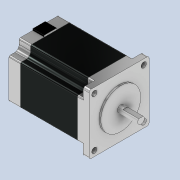
# Autodesk Inventor part: Nema 23 76.5mm Stepper Motor
Saved by Autodesk Inventor 2022 (Build 260153000, 153)
## iProperties
Created: 2021-10-18
Part Number: Nema 23 76.5mm Stepper Motor
Material: Generic
Document SubType Name: Modeling
Designer: Coy
Density: 1 g/cm^3
Appearance: Chrome - Polished
Author: Coy
Autodesk Inventor part; units mm, degrees
ref_plane "YZ Plane" through (0, 0, 0) normal (1, 0, 0) x (0, 1, 0)
ref_plane "XZ Plane" through (0, 0, 0) normal (0, 1, 0) x (-1, 0, 0)
ref_plane "XY Plane" through (0, 0, 0) normal (0, 0, 1) x (1, 0, 0)
sketch "Sketch1" plane through (0, 0, 0) normal (1, 0, 0) x (0, 1, 0)
  line L0 (2, 0) -> (55.3, 0)
  line L1 (57.3, -2) -> (57.3, -55.3)
  line L2 (55.3, -57.3) -> (2, -57.3)
  line L3 (0, -55.3) -> (0, -2)
  arc A0 (57.3, -2) -> (55.3, 0) centre (55.3, -2) ccw
  arc A1 (55.3, -57.3) -> (57.3, -55.3) centre (55.3, -55.3) ccw
  arc A2 (0, -55.3) -> (2, -57.3) centre (2, -55.3) ccw
  arc A3 (2, 0) -> (0, -2) centre (2, -2) ccw
  line L4 (52.22, -5.08) -> (5.08, -5.08) construction
  line L5 (5.08, -5.08) -> (5.08, -52.22) construction
  line L6 (5.08, -52.22) -> (52.22, -52.22) construction
  line L7 (52.22, -52.22) -> (52.22, -5.08) construction
  line L8 (52.22, -5.08) -> (57.3, -5.08) construction
  line L9 (52.22, -5.08) -> (52.22, 0) construction
  line L10 (5.08, -52.22) -> (0, -52.22) construction
  line L11 (5.08, -52.22) -> (5.08, -57.3) construction
  circle A4 centre (52.22, -5.08) radius 2.5
  circle A5 centre (52.22, -52.22) radius 2.5
  circle A6 centre (5.08, -52.22) radius 2.5
  circle A7 centre (5.08, -5.08) radius 2.5
  point P0 (0, 0)
  point P1 (57.3, -57.3)
  point P2 (57.3, 0)
  point P3 (0, -57.3)
  dimension "d0" = 57.3
  dimension "d1" = 57.3
  dimension "d2" = 2
  dimension "d3" = 2
  dimension "d4" = 5
  dimension "d5" = 5
  dimension "d6" = 5
  dimension "d7" = 5
  dimension "d8" = 47.14
  dimension "d9" = 47.14
  constraints: 24 end point, 12 point on line, 8 centre point, 8 point on circle, 8 tangent, 6 parallel, 6 perpendicular, 4 coincident, 2 equal radius, 2 horizontal
  measures "d0" distance of point (57.3, -57.3) point (0, -57.3)
  measures "d1" distance of point (57.3, 0) point (57.3, -57.3)
  measures "d2" radius of A0
  measures "d3" radius of A3
  measures "d4" diameter of A4
  measures "d5" diameter of A5
  measures "d6" diameter of A6
  measures "d7" diameter of A7
  measures "d8" distance of L4.start L4.end
  measures "d9" distance of L6.end L4.start
extrude "Extrusion1" add sketch "Sketch1" along normal blind 5.5
sketch "Sketch2" plane through (0, 0, 0) normal (-1, 0, 0) x (0, 0, 1)
  line L0 (-57.3, 2) -> (-57.3, 55.3) construction
  arc A0 (-57.3, 2) -> (-55.3, 0) centre (-55.3, 2) ccw projected
  line L1 (-2, 0) -> (-55.3, 0) construction
  arc A1 (-2, 0) -> (0, 2) centre (-2, 2) ccw projected
  line L2 (0, 55.3) -> (0, 2) construction
  arc A2 (0, 55.3) -> (-2, 57.3) centre (-2, 55.3) ccw projected
  line L3 (-55.3, 57.3) -> (-2, 57.3) construction
  arc A3 (-55.3, 57.3) -> (-57.3, 55.3) centre (-55.3, 55.3) ccw projected
  circle A4 centre (-5.08, 52.22) radius 2.5 projected
  circle A5 centre (-52.22, 52.22) radius 2.5 projected
  circle A6 centre (-52.22, 5.08) radius 2.5 projected
  circle A7 centre (-5.08, 5.08) radius 2.5 projected
  line L4 (-55.3, 57.3) -> (-2, 57.3) construction
  line L5 (-47.65, 57.3) -> (-9.65, 57.3)
  line L6 (-57.3, 2) -> (-57.3, 55.3) construction
  line L7 (-57.3, 9.65) -> (-57.3, 47.65)
  line L8 (-2, 0) -> (-55.3, 0) construction
  line L9 (-47.65, 0) -> (-9.65, 0)
  line L10 (0, 9.65) -> (0, 47.65)
  line L11 (0, 55.3) -> (0, 2) construction
  circle A8 centre (-52.22, 5.08) radius 2.5 construction
  line L12 (-52.22, 5.08) -> (-5.08, 52.22) construction
  line L13 (-28.65, 28.65) -> (-28.65, 57.3) construction
  line L14 (-28.65, 28.65) -> (-28.65, 0) construction
  line L15 (-28.65, 28.65) -> (0, 28.65) construction
  line L16 (-28.65, 28.65) -> (-57.3, 28.65) construction
  arc A9 (-51.5421, 47.65) -> (-47.6, 52.22) centre (-52.22, 52.22) ccw
  arc A10 (-9.7, 52.22) -> (-5.7579, 47.65) centre (-5.08, 52.22) ccw
  arc A11 (-5.7579, 9.65) -> (-9.7, 5.08) centre (-5.08, 5.08) ccw
  arc A12 (-47.6, 5.08) -> (-51.5421, 9.65) centre (-52.22, 5.08) ccw
  line L17 (-47.65, 57.3) -> (-47.6, 52.22)
  line L18 (-57.3, 47.65) -> (-51.5421, 47.65)
  line L19 (-9.7, 5.08) -> (-9.65, 0)
  line L20 (0, 9.65) -> (-5.7579, 9.65)
  line L21 (-9.6451, 47.6951) -> (-9.6048, 47.6952)
  line L22 (-5.7579, 47.65) -> (0, 47.65)
  line L23 (-9.65, 57.3) -> (-9.7, 52.22)
  line L24 (-9.6451, 47.6951) -> (-9.6451, 47.6549)
  line L25 (-47.6048, 9.6549) -> (-47.6452, 9.6548)
  line L26 (-51.5421, 9.65) -> (-57.3, 9.65)
  line L27 (-47.6049, 9.6951) -> (-47.6048, 9.6549)
  line L28 (-47.6, 5.08) -> (-47.65, 0)
  arc A13 (-56.05, 47.65) -> (-57.3, 46.4) centre (-56.05, 46.4) ccw
  arc A14 (-46.3876, 57.3) -> (-47.6376, 56.0377) centre (-46.3876, 56.05) ccw
  arc A15 (-9.6624, 56.0377) -> (-10.9124, 57.3) centre (-10.9124, 56.05) ccw
  arc A16 (0, 46.4) -> (-1.25, 47.65) centre (-1.25, 46.4) ccw
  arc A17 (-1.25, 9.65) -> (0, 10.9) centre (-1.25, 10.9) ccw
  arc A18 (-10.9124, 0) -> (-9.6624, 1.2623) centre (-10.9124, 1.25) ccw
  arc A19 (-47.6376, 1.2623) -> (-46.3876, 0) centre (-46.3876, 1.25) ccw
  arc A20 (-57.3, 10.9) -> (-56.05, 9.65) centre (-56.05, 10.9) ccw
  line L29 (-55.3, 57.3) -> (-2, 57.3) projected
  line L30 (-57.3, 2) -> (-57.3, 55.3) projected
  line L31 (0, 55.3) -> (0, 2) projected
  point P0 (0, 0)
  point P1 (-10.9124, 57.3)
  dimension "d12" = 38
  dimension "d13" = 38
  dimension "d14" = 38
  dimension "d15" = 38
  dimension "d16" = 2.12
  dimension "d17" = 2.12
  dimension "d18" = 2.12
  dimension "d19" = 2.12
  dimension "d20" = 2.5
  dimension "d21" = 2.5
  dimension "d22" = 2.5
  dimension "d23" = 2.5
  dimension "d24" = 2.5
  dimension "d25" = 2.5
  dimension "d26" = 2.5
  dimension "d27" = 2.5
  constraints: 42 end point, 27 point on line, 24 point on circle, 16 tangent, 12 centre point, 5 midpoint, 3 vertical, 2 horizontal
  measures "d12" distance of L5.start L5.end
  measures "d13" distance of L7.start L7.end
  measures "d14" distance of L10.end L10.start
  measures "d15" distance of L9.start L9.end
  measures "d16" radial gap between concentric circles of A5 A9
  measures "d17" radial gap between concentric circles of A4 A10
  measures "d18" radial gap between concentric circles of A7 A11
  measures "d19" radial gap between concentric circles of A6 A12
  measures "d20" diameter of A13
  measures "d21" diameter of A14
  measures "d22" diameter of A15
  measures "d23" diameter of A16
  measures "d24" diameter of A17
  measures "d25" diameter of A18
  measures "d26" diameter of A19
  measures "d27" diameter of A20
extrude "Extrusion2" add sketch "Sketch2" along normal blind 5.5 contours L10 A17 L20 A11 L19 A18 L9 A19 L28 A12 L26 A20 L7 A13 L18 A9 L17 A14 L5 A15 L23 A10 L22 A16
sketch "Sketch3" plane through (-5.5, 0, 0) normal (-1, 0, 0) x (0, 0, 1)
  line L0 (-51.5421, 47.65) -> (-56.05, 47.65) projected
  arc A0 (-56.05, 47.65) -> (-57.3, 46.4) centre (-56.05, 46.4) ccw projected
  line L1 (-57.3, 46.4) -> (-57.3, 10.9) projected
  arc A1 (-57.3, 10.9) -> (-56.05, 9.65) centre (-56.05, 10.9) ccw projected
  line L2 (-56.05, 9.65) -> (-51.5421, 9.65) projected
  arc A2 (-47.6, 5.08) -> (-51.5421, 9.65) centre (-52.22, 5.08) ccw projected
  line L3 (-47.6, 5.08) -> (-47.6376, 1.2623) projected
  arc A3 (-47.6376, 1.2623) -> (-46.3876, 0) centre (-46.3876, 1.25) ccw projected
  line L4 (-46.3876, 0) -> (-10.9124, 0) projected
  arc A4 (-10.9124, 0) -> (-9.6624, 1.2623) centre (-10.9124, 1.25) ccw projected
  line L5 (-9.6624, 1.2623) -> (-9.7, 5.08) projected
  arc A5 (-5.7579, 9.65) -> (-9.7, 5.08) centre (-5.08, 5.08) ccw projected
  line L6 (-5.7579, 9.65) -> (-1.25, 9.65) projected
  arc A6 (-1.25, 9.65) -> (0, 10.9) centre (-1.25, 10.9) ccw projected
  line L7 (0, 10.9) -> (0, 46.4) projected
  arc A7 (0, 46.4) -> (-1.25, 47.65) centre (-1.25, 46.4) ccw projected
  line L8 (-1.25, 47.65) -> (-5.7579, 47.65) projected
  arc A8 (-9.7, 52.22) -> (-5.7579, 47.65) centre (-5.08, 52.22) ccw projected
  line L9 (-9.7, 52.22) -> (-9.6624, 56.0377) projected
  arc A9 (-9.6624, 56.0377) -> (-10.9124, 57.3) centre (-10.9124, 56.05) ccw projected
  line L10 (-10.9124, 57.3) -> (-46.3876, 57.3) projected
  arc A10 (-46.3876, 57.3) -> (-47.6376, 56.0377) centre (-46.3876, 56.05) ccw projected
  line L11 (-47.6376, 56.0377) -> (-47.6, 52.22) projected
  arc A11 (-51.5421, 47.65) -> (-47.6, 52.22) centre (-52.22, 52.22) ccw projected
  line L12 (-46.3876, 57.2) -> (-10.9124, 57.2)
  arc A12 (-9.7624, 56.0387) -> (-10.9124, 57.2) centre (-10.9124, 56.05) ccw
  line L13 (-9.7624, 56.0387) -> (-9.8, 52.2205)
  arc A13 (-9.8, 52.2205) -> (-5.7652, 47.55) centre (-5.08, 52.22) ccw
  line L14 (-5.7652, 47.55) -> (-1.25, 47.55)
  arc A14 (-0.1, 46.4) -> (-1.25, 47.55) centre (-1.25, 46.4) ccw
  line L15 (-0.1, 46.4) -> (-0.1, 10.9)
  arc A15 (-1.25, 9.75) -> (-0.1, 10.9) centre (-1.25, 10.9) ccw
  line L16 (-1.25, 9.75) -> (-5.7652, 9.75)
  arc A16 (-5.7652, 9.75) -> (-9.8, 5.0795) centre (-5.08, 5.08) ccw
  line L17 (-9.8, 5.0795) -> (-9.7624, 1.2613)
  arc A17 (-10.9124, 0.1) -> (-9.7624, 1.2613) centre (-10.9124, 1.25) ccw
  line L18 (-10.9124, 0.1) -> (-46.3876, 0.1)
  arc A18 (-47.5376, 1.2613) -> (-46.3876, 0.1) centre (-46.3876, 1.25) ccw
  line L19 (-47.5376, 1.2613) -> (-47.5, 5.0795)
  arc A19 (-47.5, 5.0795) -> (-51.5348, 9.75) centre (-52.22, 5.08) ccw
  line L20 (-51.5348, 9.75) -> (-56.05, 9.75)
  arc A20 (-57.2, 10.9) -> (-56.05, 9.75) centre (-56.05, 10.9) ccw
  line L21 (-57.2, 10.9) -> (-57.2, 46.4)
  arc A21 (-56.05, 47.55) -> (-57.2, 46.4) centre (-56.05, 46.4) ccw
  line L22 (-56.05, 47.55) -> (-51.5348, 47.55)
  arc A22 (-51.5348, 47.55) -> (-47.5, 52.2205) centre (-52.22, 52.22) ccw
  line L23 (-47.5, 52.2205) -> (-47.5376, 56.0387)
  arc A23 (-46.3876, 57.2) -> (-47.5376, 56.0387) centre (-46.3876, 56.05) ccw
  point P0 (0, 0)
  dimension "d30" = 0.1
  constraints: 24 end point, 24 point on circle, 12 centre point, 23 other
  measures "d30" distance between parallel lines of L10 L12
extrude "Extrusion3" add sketch "Sketch3" along normal blind 54.5 contours L12 A12 L13 A13 L14 A14 L15 A15 L16 A16 L17 A17 L18 A18 L19 A19 L20 A20 L21 A21 L22 A22 L23 A23
sketch "Sketch4" plane through (-60, 0, 0) normal (-1, 0, 0) x (0, 0, 1)
  arc A0 (-56.05, 47.55) -> (-57.2, 46.4) centre (-56.05, 46.4) ccw projected
  line L0 (-56.05, 47.55) -> (-51.5348, 47.55) projected
  arc A1 (-51.5348, 47.55) -> (-47.5, 52.2205) centre (-52.22, 52.22) ccw projected
  line L1 (-47.5, 52.2205) -> (-47.5376, 56.0387) projected
  arc A2 (-46.3876, 57.2) -> (-47.5376, 56.0387) centre (-46.3876, 56.05) ccw projected
  line L2 (-46.3876, 57.2) -> (-10.9124, 57.2) projected
  arc A3 (-9.7624, 56.0387) -> (-10.9124, 57.2) centre (-10.9124, 56.05) ccw projected
  line L3 (-9.7624, 56.0387) -> (-9.8, 52.2205) projected
  arc A4 (-9.8, 52.2205) -> (-5.7652, 47.55) centre (-5.08, 52.22) ccw projected
  line L4 (-5.7652, 47.55) -> (-1.25, 47.55) projected
  arc A5 (-0.1, 46.4) -> (-1.25, 47.55) centre (-1.25, 46.4) ccw projected
  line L5 (-0.1, 46.4) -> (-0.1, 10.9) projected
  arc A6 (-1.25, 9.75) -> (-0.1, 10.9) centre (-1.25, 10.9) ccw projected
  line L6 (-1.25, 9.75) -> (-5.7652, 9.75) projected
  arc A7 (-5.7652, 9.75) -> (-9.8, 5.0795) centre (-5.08, 5.08) ccw projected
  line L7 (-9.8, 5.0795) -> (-9.7624, 1.2613) projected
  arc A8 (-10.9124, 0.1) -> (-9.7624, 1.2613) centre (-10.9124, 1.25) ccw projected
  line L8 (-10.9124, 0.1) -> (-46.3876, 0.1) projected
  arc A9 (-47.5376, 1.2613) -> (-46.3876, 0.1) centre (-46.3876, 1.25) ccw projected
  line L9 (-47.5376, 1.2613) -> (-47.5, 5.0795) projected
  arc A10 (-47.5, 5.0795) -> (-51.5348, 9.75) centre (-52.22, 5.08) ccw projected
  line L10 (-51.5348, 9.75) -> (-56.05, 9.75) projected
  arc A11 (-57.2, 10.9) -> (-56.05, 9.75) centre (-56.05, 10.9) ccw projected
  line L11 (-57.2, 10.9) -> (-57.2, 46.4) projected
  line L12 (-51.5421, 47.65) -> (-56.05, 47.65) projected
  arc A12 (-56.05, 47.65) -> (-57.3, 46.4) centre (-56.05, 46.4) ccw projected
  line L13 (-57.3, 46.4) -> (-57.3, 10.9) projected
  arc A13 (-57.3, 10.9) -> (-56.05, 9.65) centre (-56.05, 10.9) ccw projected
  line L14 (-56.05, 9.65) -> (-51.5421, 9.65) projected
  arc A14 (-47.6, 5.08) -> (-51.5421, 9.65) centre (-52.22, 5.08) ccw projected
  line L15 (-47.6, 5.08) -> (-47.6376, 1.2623) projected
  arc A15 (-47.6376, 1.2623) -> (-46.3876, 0) centre (-46.3876, 1.25) ccw projected
  line L16 (-46.3876, 0) -> (-10.9124, 0) projected
  arc A16 (-10.9124, 0) -> (-9.6624, 1.2623) centre (-10.9124, 1.25) ccw projected
  line L17 (-9.6624, 1.2623) -> (-9.7, 5.08) projected
  arc A17 (-5.7579, 9.65) -> (-9.7, 5.08) centre (-5.08, 5.08) ccw projected
  line L18 (-5.7579, 9.65) -> (-1.25, 9.65) projected
  arc A18 (-1.25, 9.65) -> (0, 10.9) centre (-1.25, 10.9) ccw projected
  line L19 (0, 10.9) -> (0, 46.4) projected
  arc A19 (0, 46.4) -> (-1.25, 47.65) centre (-1.25, 46.4) ccw projected
  line L20 (-1.25, 47.65) -> (-5.7579, 47.65) projected
  arc A20 (-9.7, 52.22) -> (-5.7579, 47.65) centre (-5.08, 52.22) ccw projected
  line L21 (-9.7, 52.22) -> (-9.6624, 56.0377) projected
  arc A21 (-9.6624, 56.0377) -> (-10.9124, 57.3) centre (-10.9124, 56.05) ccw projected
  line L22 (-10.9124, 57.3) -> (-46.3876, 57.3) projected
  arc A22 (-46.3876, 57.3) -> (-47.6376, 56.0377) centre (-46.3876, 56.05) ccw projected
  line L23 (-47.6376, 56.0377) -> (-47.6, 52.22) projected
  arc A23 (-51.5421, 47.65) -> (-47.6, 52.22) centre (-52.22, 52.22) ccw projected
  point P0 (0, 0)
extrude "Extrusion4" add sketch "Sketch4" along normal blind 11 contours L0 A1 L1 A2 L2 A3 L3 A4 L4 A5 L5 A6 L6 A7 L7 A8 L8 A9 L9 A10 L10 A11 L11 A0 | A23 L23 A22 L22 A21 L21 A20 L20 A19 L19 A18 L18 A17 L17 A16 L16 A15 L15 A14 L14 A13 L13 A12 L12
sketch "Sketch5" plane through (5.5, 0, 0) normal (1, 0, 0) x (0, 0, -1)
  line L0 (46.3876, 57.2) -> (10.9124, 57.2) construction
  line L1 (28.65, 57.2) -> (28.65, 0.1) construction
  line L2 (10.9124, 0.1) -> (46.3876, 0.1) construction
  circle A0 centre (28.65, 28.65) radius 19.05
  point P0 (0, 0)
  dimension "d35" = 38.1
  constraints: 3 midpoint, 2 end point, 1 centre point
  measures "d35" diameter of A0
extrude "Extrusion5" add sketch "Sketch5" along normal blind 1.6
sketch "Sketch6" plane through (7.1, 28.65, -28.65) normal (1, 0, 0) x (0, 0, -1)
  circle A0 centre (0, 0) radius 3.175
  point P0 (-28.65, -28.65)
  dimension "d38" = 6.35
  constraints: 1 centre point
  measures "d38" diameter of A0
extrude "Extrusion6" add sketch "Sketch6" along normal blind 4.4
sketch "Sketch7" plane through (11.5, 28.65, -28.65) normal (1, 0, 0) x (0, 0, -1)
  circle A0 centre (0, 0) radius 3.175 projected
  line L0 (-9.5378, 2.375) -> (9.1058, 2.375)
  point P0 (-28.65, -28.65)
  point P1 (2.1071, 2.375)
  point P2 (-2.1071, 2.375)
  dimension "d41" = 2.375
  constraints: 2 end point, 1 horizontal
  measures "d41" distance from line of A0.centre L0
extrude "Extrusion7" add sketch "Sketch7" along normal blind 15 contours A0 L0 picked at (0.5748, 0.6947)
sketch "Sketch8" plane through (-60, 57.3, -10.9124) normal (0, 1, 0) x (1, 0, 0)
  line L0 (-11, 35.4753) -> (-11, 0) projected
  line L1 (0, 0) -> (0, 35.4753) projected
  line L2 (-11, 11.75) -> (0, 11.75)
  line L3 (0, 11.75) -> (0, 23.75)
  line L4 (0, 23.75) -> (-11, 23.75)
  line L5 (-11, 23.75) -> (-11, 11.75)
  point P0 (60, -10.9124)
  point P1 (-11, 23.75)
  point P2 (0, 11.75)
  dimension "d44" = 12
  dimension "d45" = 11.75
  constraints: 8 end point, 2 parallel, 2 point on line, 1 horizontal, 1 perpendicular
  measures "d44" distance of L3.end L2.end
  measures "d45" distance from line of L0.end L2
extrude "Extrusion8" add sketch "Sketch8" along normal blind 1.5
equation "\"d5\" = d4"
equation "\"d6\" = d4"
equation "\"d7\" = d4"
equation "\"d13\" = d12"
equation "\"d14\" = d12"
equation "\"d15\" = d12"
equation "\"d17\" = d16"
equation "\"d18\" = d16"
equation "\"d19\" = d16"
equation "\"d21\" = d20"
equation "\"d22\" = d20"
equation "\"d23\" = d20"
equation "\"d24\" = d20"
equation "\"d25\" = d20"
equation "\"d26\" = d20"
equation "\"d27\" = d20"
body "Solid1"
